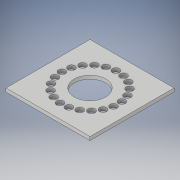
# Autodesk Inventor part: basePlate
Saved by Autodesk Inventor 2019 (Build 230136000, 136)
## iProperties
Created: 2019-05-17
Part Number: basePlate
Material: Generic
Document SubType Name: Modeling
Designer: Alex Jones
Density: 1 g/cm^3
Appearance: Default
Author: Alex Jones
Autodesk Inventor part; units mm, degrees
ref_plane "YZ Plane" through (0, 0, 0) normal (1, 0, 0) x (0, 1, 0)
ref_plane "XZ Plane" through (0, 0, 0) normal (0, 1, 0) x (-1, 0, 0)
ref_plane "XY Plane" through (0, 0, 0) normal (0, 0, 1) x (1, 0, 0)
sketch "Sketch1" plane through (0, 0, 0) normal (0, 1, 0) x (-1, 0, 0)
  circle A0 centre (0, 0) radius 25.4 construction
  circle A1 centre (25.4, 0) radius 3.175
  line L0 (-38.1, 38.1) -> (38.1, 38.1)
  line L1 (38.1, 38.1) -> (38.1, -38.1)
  line L2 (38.1, -38.1) -> (-38.1, -38.1)
  line L3 (-38.1, -38.1) -> (-38.1, 38.1)
  line L4 (-38.1, 38.1) -> (38.1, -38.1) construction
  line L5 (38.1, 38.1) -> (-38.1, -38.1) construction
  circle A2 centre (24.2715, -7.4868) radius 3.175
  circle A3 centre (20.9865, -14.3083) radius 3.175
  circle A4 centre (15.8366, -19.8585) radius 3.175
  circle A5 centre (9.2797, -23.6442) radius 3.175
  circle A6 centre (1.8981, -25.329) radius 3.175
  circle A7 centre (-5.652, -24.7632) radius 3.175
  circle A8 centre (-12.7, -21.997) radius 3.175
  circle A9 centre (-18.6195, -17.2764) radius 3.175
  circle A10 centre (-22.8846, -11.0206) radius 3.175
  circle A11 centre (-25.1163, -3.7857) radius 3.175
  circle A12 centre (-25.1163, 3.7857) radius 3.175
  circle A13 centre (-22.8846, 11.0206) radius 3.175
  circle A14 centre (-18.6195, 17.2764) radius 3.175
  circle A15 centre (-12.7, 21.997) radius 3.175
  circle A16 centre (-5.652, 24.7632) radius 3.175
  circle A17 centre (1.8981, 25.329) radius 3.175
  circle A18 centre (9.2797, 23.6442) radius 3.175
  circle A19 centre (15.8366, 19.8585) radius 3.175
  circle A20 centre (20.9865, 14.3083) radius 3.175
  circle A21 centre (24.2715, 7.4868) radius 3.175
  circle A22 centre (0, 0) radius 14.25
  dimension "d0" = 50.8
  dimension "d1" = 6.35
  dimension "d6" = 76.2
  dimension "d7" = 76.2
  dimension "d15" = 360
  dimension "d17" = 28.5
  constraints: 22 centre point, 12 end point, 2 coincident, 2 midpoint, 2 parallel, 1 horizontal, 1 horizontal alignment, 1 perpendicular, 45 other
  measures "d1" diameter of A1
  measures "d6" distance of L1.end L2.end
  measures "d7" distance of L0.end L1.end
  measures "d17" diameter of A22
extrude "Extrusion1" add sketch "Sketch1" along normal blind 3.175
body "Solid1"
